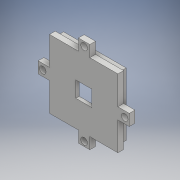
# Autodesk Inventor part: LidClampCell_V6
Saved by Autodesk Inventor 2018 (Build 220112000, 112)
## iProperties
Created: 2018-06-07
Part Number: LidClampCell_V6
Material: Generic
Document SubType Name: Modeling
Designer: Anna Dorfi
Density: 1 g/cm^3
Appearance: Default
Author: Anna Dorfi
Autodesk Inventor part; units mm, degrees
ref_plane "YZ Plane" through (0, 0, 0) normal (1, 0, 0) x (0, 1, 0)
ref_plane "XZ Plane" through (0, 0, 0) normal (0, 1, 0) x (-1, 0, 0)
ref_plane "XY Plane" through (0, 0, 0) normal (0, 0, 1) x (1, 0, 0)
sketch "Sketch1" plane through (0, 0, 0) normal (0, 1, 0) x (-1, 0, 0)
  circle A0 centre (28.1298, -0.9274) radius 1
  circle A1 centre (3.1298, -25.9274) radius 1
  circle A2 centre (-21.8702, -0.9274) radius 1
  circle A3 centre (3.1298, 24.0726) radius 1
  line L0 (33.1298, -30.9274) -> (-26.8702, -30.9274)
  line L1 (-26.8702, -30.9274) -> (-26.8702, 29.0726)
  line L2 (-26.8702, 29.0726) -> (33.1298, 29.0726)
  line L3 (33.1298, 29.0726) -> (33.1298, -30.9274)
  line L4 (33.1298, -30.9274) -> (-26.8702, 29.0726) construction
  line L5 (-26.8702, -30.9274) -> (33.1298, 29.0726) construction
  point P0 (0, 0)
  dimension "d1" = 2
  dimension "d2" = 2
  dimension "d3" = 2
  dimension "d4" = 2
  dimension "d7" = 60
  dimension "d9" = 50
  dimension "d10" = 50
  dimension "d12" = 5
  dimension "d13" = 60
  dimension "d14" = 5
  dimension "d15" = 30
  dimension "d16" = 30
  dimension "d17" = 30
  constraints: 12 end point, 4 centre point, 2 parallel, 1 horizontal, 1 perpendicular
  measures "d1" diameter of A0
  measures "d2" diameter of A1
  measures "d3" diameter of A2
  measures "d4" diameter of A3
  measures "d7" distance of L2.end L0.start
  measures "d9" distance of A3.centre A1.centre
  measures "d10" distance of A0.centre A2.centre
  measures "d12" distance from line of A1.centre L0
  measures "d13" distance of L1.end L2.end
  measures "d14" distance from line of L3 A0.centre
  measures "d15" distance from line of L2 A0.centre
  measures "d16" distance from line of L2 A2.centre
  measures "d17" distance from line of L1 A1.centre
extrude "Extrusion1" add sketch "Sketch1" along normal blind 5 contours A0 | A1 | A2 | A3 | L0 L1 L2 L3
sketch "Sketch2" plane through (0, 5, 0) normal (0, 1, 0) x (1, 0, 0)
  line L0 (26.8702, 30.9274) -> (-33.1298, 30.9274) projected
  line L1 (-7.7791, 30.9274) -> (2.2209, 30.9274)
  line L2 (2.2209, 30.9274) -> (2.2209, 40.9274)
  line L3 (2.2209, 40.9274) -> (-7.7791, 40.9274)
  line L4 (-7.7791, 40.9274) -> (-7.7791, 30.9274)
  line L5 (-33.1298, -29.0726) -> (26.8702, -29.0726) projected
  line L6 (-7.7791, -29.0726) -> (2.2209, -29.0726)
  line L7 (2.2209, -29.0726) -> (2.2209, -39.0726)
  line L8 (2.2209, -39.0726) -> (-7.7791, -39.0726)
  line L9 (-7.7791, -39.0726) -> (-7.7791, -29.0726)
  point P0 (0, 0)
  dimension "d18" = 10
  dimension "d19" = 10
  dimension "d20" = 10
  constraints: 16 end point, 4 parallel, 4 point on line, 2 horizontal, 2 perpendicular
  measures "d18" distance of L3.end L2.end
  measures "d19" distance of L8.end L6.start
  measures "d20" distance of L3.end L1.start
extrude "Extrusion2" add sketch "Sketch2" against normal blind 5
sketch "Sketch3" plane through (0, 0, 0) normal (0, -1, 0) x (1, 0, 0)
  circle A0 centre (-2.7791, -36.9274) radius 2.925
  circle A1 centre (-2.7791, 35.0726) radius 2.925
  line L0 (-7.7791, 39.0726) -> (-7.7791, 29.0726) projected
  line L1 (2.2209, 39.0726) -> (-7.7791, 39.0726) projected
  line L2 (-7.7791, -40.9274) -> (2.2209, -40.9274) projected
  line L3 (-7.7791, -30.9274) -> (-7.7791, -40.9274) projected
  point P0 (0, 0)
  dimension "d23" = 5.85
  dimension "d24" = 5.85
  dimension "d25" = 5
  dimension "d26" = 4
  dimension "d27" = 4
  dimension "d28" = 5
  constraints: 2 centre point
  measures "d23" diameter of A0
  measures "d24" diameter of A1
  measures "d25" distance from line of L0 A1.centre
  measures "d26" distance from line of L1 A1.centre
  measures "d27" distance from line of L2 A0.centre
  measures "d28" distance from line of L3 A0.centre
extrude "Extrusion3" cut sketch "Sketch3" along normal through all both and the other way through all
sketch "Sketch4" plane through (0, 0, 0) normal (0, -1, 0) x (1, 0, 0)
  line L0 (-10.1298, 6.0726) -> (3.8702, 6.0726)
  line L1 (3.8702, 6.0726) -> (3.8702, -7.9274)
  line L2 (3.8702, -7.9274) -> (-10.1298, -7.9274)
  line L3 (-10.1298, -7.9274) -> (-10.1298, 6.0726)
  line L4 (-33.1298, 29.0726) -> (-33.1298, -30.9274) projected
  line L5 (26.8702, -30.9274) -> (26.8702, 29.0726) projected
  line L6 (-33.1298, -30.9274) -> (-7.7791, -30.9274) projected
  line L7 (26.8702, 29.0726) -> (-33.1298, 29.0726) projected
  point P0 (0, 0)
  point P1 (-7.7791, 29.0726)
  dimension "d31" = 14
  dimension "d32" = 14
  dimension "d33" = 23
  dimension "d34" = 23
  dimension "d35" = 23
  dimension "d36" = 23
  constraints: 8 end point, 2 parallel, 1 horizontal, 1 perpendicular
  measures "d31" distance of L1.end L2.end
  measures "d32" distance of L0.end L1.end
  measures "d33" distance between parallel lines of L4 L3
  measures "d34" distance between parallel lines of L5 L1
  measures "d35" distance between parallel lines of L6 L2
  measures "d36" distance between parallel lines of L7 L0
extrude "Extrusion4" cut sketch "Sketch4" against normal through all
sketch "Sketch5" plane through (0, 5, 0) normal (0, 1, 0) x (1, 0, 0)
  line L0 (-43.1298, -4.0726) -> (-33.1298, -4.0726)
  line L1 (-33.1298, -4.0726) -> (-33.1298, 5.9274)
  line L2 (-33.1298, 5.9274) -> (-43.1298, 5.9274)
  line L3 (-43.1298, 5.9274) -> (-43.1298, -4.0726)
  line L4 (-33.1298, -29.0726) -> (-7.7791, -29.0726) projected
  line L5 (-33.1298, 30.9274) -> (-33.1298, -29.0726) projected
  line L6 (26.8702, 30.9274) -> (26.8702, -29.0726) projected
  line L7 (26.8702, -4.0726) -> (36.8702, -4.0726)
  line L8 (36.8702, -4.0726) -> (36.8702, 5.9274)
  line L9 (36.8702, 5.9274) -> (26.8702, 5.9274)
  line L10 (26.8702, 5.9274) -> (26.8702, -4.0726)
  line L11 (26.8702, 30.9274) -> (2.2209, 30.9274) projected
  line L12 (2.2209, -29.0726) -> (26.8702, -29.0726) projected
  line L13 (26.8702, -29.0726) -> (26.8702, 30.9274) projected
  point P0 (0, 0)
  dimension "d39" = 10
  dimension "d40" = 10
  dimension "d41" = 25
  dimension "d42" = 0
  dimension "d43" = 10
  dimension "d44" = 10
  dimension "d45" = 25
  dimension "d46" = 25
  dimension "d47" = 10
  constraints: 16 end point, 4 parallel, 2 horizontal, 2 perpendicular, 1 point on line
  measures "d39" distance of L2.end L1.end
  measures "d40" distance of L1.end L0.end
  measures "d41" distance between parallel lines of L4 L0
  measures "d42" distance between parallel lines of L5 L1
  measures "d43" distance of L9.end L8.end
  measures "d44" distance of L8.end L7.end
  measures "d45" distance between parallel lines of L11 L9
  measures "d46" distance between parallel lines of L12 L7
  measures "d47" distance between parallel lines of L13 L8
extrude "Extrusion5" add sketch "Sketch5" against normal blind 5
sketch "Sketch6" plane through (0, 5, 0) normal (0, 1, 0) x (1, 0, 0)
  circle A0 centre (-39.1298, 0.9274) radius 2.925
  circle A1 centre (32.8702, 0.9274) radius 2.925
  line L0 (36.8702, 5.9274) -> (26.8702, 5.9274) projected
  line L1 (26.8702, -29.0726) -> (26.8702, -4.0726) projected
  line L2 (36.8702, -4.0726) -> (36.8702, 5.9274) projected
  line L3 (-43.1298, 5.9274) -> (-43.1298, -4.0726) projected
  line L4 (-33.1298, 5.9274) -> (-43.1298, 5.9274) projected
  point P0 (0, 0)
  dimension "d50" = 5.85
  dimension "d51" = 5.85
  dimension "d52" = 5
  dimension "d54" = 4
  dimension "d55" = 4
  dimension "d56" = 5
  constraints: 2 centre point
  measures "d50" diameter of A0
  measures "d51" diameter of A1
  measures "d52" distance from line of L0 A1.centre
  measures "d54" distance from line of L2 A1.centre
  measures "d55" distance from line of L3 A0.centre
  measures "d56" distance from line of L4 A0.centre
extrude "Extrusion6" cut sketch "Sketch6" against normal through all
sketch "Sketch7" plane through (0, 5, 0) normal (0, 1, 0) x (1, 0, 0)
  line L0 (-24.9285, -19.3498) -> (16.3215, -19.3498)
  line L1 (16.3215, -19.3498) -> (16.3215, 21.9002)
  line L2 (16.3215, 21.9002) -> (-24.9285, 21.9002)
  line L3 (-24.9285, 21.9002) -> (-24.9285, -19.3498)
  line L4 (-33.1298, -29.0726) -> (-7.7791, -29.0726) projected
  line L5 (26.8702, -29.0726) -> (26.8702, -4.0726) projected
  line L6 (-31.8035, -26.2248) -> (23.1965, -26.2248)
  line L7 (23.1965, -26.2248) -> (23.1965, 28.7752)
  line L8 (23.1965, 28.7752) -> (-31.8035, 28.7752)
  line L9 (-31.8035, 28.7752) -> (-31.8035, -26.2248)
  line L10 (26.8702, 30.9274) -> (2.2209, 30.9274) projected
  line L11 (2.2209, -29.0726) -> (26.8702, -29.0726) projected
  line L12 (-33.1298, -4.0726) -> (-33.1298, -29.0726) projected
  point P0 (0, 0)
  dimension "d78" = 55
  constraints: 16 end point, 4 parallel, 2 horizontal, 2 perpendicular
  measures "d78" distance of L6.end L7.end
extrude "Extrusion7" add sketch "Sketch7" along normal blind 6
sketch "Sketch8" plane through (0, 11, 0) normal (0, 1, 0) x (1, 0, 0)
  circle A0 centre (-27.9285, 11.9002) radius 0.75
  line L0 (-24.9285, -19.3498) -> (-24.9285, 21.9002) projected
  line L1 (-24.9285, 21.9002) -> (16.3215, 21.9002) projected
  point P0 (0, 0)
  dimension "d70" = 1.5
  dimension "d71" = 3
  dimension "d80" = 10
  constraints: 1 centre point
  measures "d70" diameter of A0
  measures "d71" distance from line of L0 A0.centre
  measures "d80" distance from line of L1 A0.centre
sketch "Sketch9" plane through (-24.9285, 5, 19.3498) normal (1, 0, 0) x (0, 0, -1)
  circle A0 centre (31.25, 2.5) radius 0.75
  line L0 (0, 6) -> (41.25, 6) projected
  point P0 (19.3498, -5)
  dimension "d72" = 1.5
  dimension "d73" = 3.5
  dimension "d81" = 10
  constraints: 1 centre point
  measures "d72" diameter of A0
  measures "d73" distance from line of L0 A0.centre
  measures "d81" horizontal distance of L0.end A0.centre
loft "Loft1" cut profiles "Sketch9", "Sketch8"
sketch "Sketch10" plane through (0, 11, 0) normal (0, 1, 0) x (1, 0, 0)
  circle A0 centre (-28.4285, -12.1344) radius 1.75
  line L0 (-24.9285, -19.3498) -> (-24.9285, 21.9002) projected
  point P0 (0, 0)
  dimension "d83" = 3.5
  dimension "d84" = 3.5
  constraints: 1 centre point
  measures "d83" diameter of A0
  measures "d84" distance from line of L0 A0.centre
sketch "Sketch11" plane through (-24.9285, 5, 19.3498) normal (1, 0, 0) x (0, 0, -1)
  circle A0 centre (6.8624, 3) radius 2
  line L0 (41.25, 0) -> (0, 0) projected
  point P0 (19.3498, -5)
  dimension "d85" = 4
  dimension "d86" = 3
  constraints: 1 centre point
  measures "d85" diameter of A0
  measures "d86" distance from line of L0 A0.centre
loft "Loft2" cut profiles "Sketch10", "Sketch11"
sketch "Sketch13" plane through (0, 5, 0) normal (0, 1, 0) x (1, 0, 0)
  line L0 (10.8215, -14.0787) -> (-17.1785, -14.0787)
  line L1 (-17.1785, -14.0787) -> (-17.1785, 15.9213)
  line L2 (-17.1785, 15.9213) -> (10.8215, 15.9213)
  line L3 (10.8215, 15.9213) -> (10.8215, -14.0787)
  line L4 (16.3215, 21.9002) -> (16.3215, -19.3498) projected
  point P0 (0, 0)
  point P1 (-12.1298, -8.0726)
  point P2 (5.8702, 9.9274)
  dimension "d104" = 30
  dimension "d105" = 28
  dimension "d106" = 5.5
  constraints: 8 end point, 2 parallel, 1 horizontal, 1 perpendicular
  measures "d104" distance of L2.end L0.start
  measures "d105" distance of L0.start L0.end
  measures "d106" distance between parallel lines of L4 L3
extrude "Extrusion9" cut sketch "Sketch13" against normal blind 2
body "Solid1"
